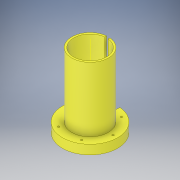
# Autodesk Inventor part: ExternalStationaryOuterRing
Saved by Autodesk Inventor 2019.3 (Build 233278000, 278)
## iProperties
Created: 2018-12-30
Part Number: ExternalStationaryOuterRing
Material: LCP Plastic
Document SubType Name: Modeling
Designer: steele
Density: 1.626 g/cm^3
Appearance: Smooth - Yellow
Author: steele
Autodesk Inventor part; units mm, degrees
ref_plane "YZ Plane" through (0, 0, 0) normal (1, 0, 0) x (0, 1, 0)
ref_plane "XZ Plane" through (0, 0, 0) normal (0, 1, 0) x (-1, 0, 0)
ref_plane "XY Plane" through (0, 0, 0) normal (0, 0, 1) x (1, 0, 0)
sketch "Sketch12" plane through (0, 0, 0) normal (0, 0, 1) x (1, 0, 0)
  line L0 (37.973, 0) -> (37.973, 12.7)
  line L1 (0, 0) -> (0, 101.6) construction
  line L2 (25.273, 101.6) -> (25.273, 12.7)
  line L3 (25.273, 12.7) -> (37.973, 12.7)
  line L4 (25.273, 101.6) -> (22.733, 101.6)
  line L5 (22.733, 101.6) -> (22.733, 0)
  line L6 (22.733, 0) -> (37.973, 0)
  line L7 (0, -20.32) -> (0, 121.92) projected
  dimension "d49" = 12.7
  dimension "d50" = 101.6
  dimension "d53" = 2.54
  dimension "d60" = 12.7
  dimension "d72" = 22.733
  constraints: 14 end point, 3 vertical, 2 parallel, 2 perpendicular, 1 horizontal
  measures "d49" distance of L0.start L0.end
  measures "d50" distance of L1.start L1.end
  measures "d53" distance of L2.start L4.end
  measures "d60" distance of L2.end L0.end
  measures "d72" distance between parallel lines of L5 L1
revolve "Revolution3" add sketch "Sketch12" angle 360 about axis through (0, 0, 0) along (0, 1, 0)
sketch "Sketch13" plane through (0, 0, 0) normal (0, -1, 0) x (1, 0, 0)
  line L0 (0, 0) -> (0, -37.973) construction
  circle A0 centre (0, 0) radius 37.973 construction
  line L1 (0, 0) -> (-3.6396, -37.7982)
  line L2 (0, 0) -> (3.6396, -37.7982)
  arc A1 (-3.6396, -37.7982) -> (3.6396, -37.7982) centre (0, 0) ccw
  dimension "d56" = 5.5
  dimension "d57" = 5.5
  constraints: 6 end point, 5 point on circle, 1 centre point, 1 coincident, 1 vertical
  measures "d56" angle of L1 L0
  measures "d57" angle of L2 L0
extrude "Extrusion5" cut sketch "Sketch13" against normal through all
sketch "Sketch17" plane through (0, 0, 0) normal (0, -1, 0) x (1, 0, 0)
  arc A0 (3.6396, -37.7982) -> (-3.6396, -37.7982) centre (0, 0) ccw projected
  point P0 (31.75, 0)
  dimension "d73" = 31.75
  measures "d73" distance of point (31.75, 0) A0.centre
hole "Hole4" at (31.75, 0, 0) direction (0, 1, 0) diameter 2.6416 end through all counterbore diameter 4.699 counterbore depth 7.1374 thread size "6-32 UNC" class "2B" standard "ANSI Unified Screw Threads"
pattern_circular "Circular Pattern2" count 6 over 360 about axis through (0, -10, 0) along (0, 1, 0) of "Hole4"
equation "\"d56\" = 0.5 * angleForSlot"
equation "\"d57\" = 0.5 * angleForSlot"
equation "\"angleForSlot\" = 11deg"
body "Solid1"
body "Solid2"
